Autodesk Fusion 360 part; units mm, degrees
(part 4 of 5)
sketch "Sketch8" plane through (0, 0, 2) normal (0, 0, 1) x (1, 0, 0)
  line L0 (-2.9765, -78.272) -> (-7.3765, -81.7096)
  arc A0 (-9.8, -80.5276) -> (-7.3765, -81.7096) centre (-8.3, -80.5276) ccw
  line L1 (-9.8, -80.5276) -> (-9.8, -73.6105)
  arc A1 (-9.1388, -72.3669) -> (-9.8, -73.6105) centre (-8.3, -73.6105) ccw
  line L2 (-9.1388, -72.3669) -> (-3.9592, -68.8733)
  arc A2 (-2.4, -69.7023) -> (-3.9592, -68.8733) centre (-3.4, -69.7023) ccw
  line L3 (-2.4, -69.7023) -> (-2.4, -77.09)
  arc A3 (-2.9765, -78.272) -> (-2.4, -77.09) centre (-3.9, -77.09) ccw
  line L4 (-2.9765, -60.272) -> (-7.3765, -63.7096)
  arc A4 (-9.8, -62.5276) -> (-7.3765, -63.7096) centre (-8.3, -62.5276) ccw
  line L5 (-9.8, -62.5276) -> (-9.8, -55.6105)
  arc A5 (-9.1388, -54.3669) -> (-9.8, -55.6105) centre (-8.3, -55.6105) ccw
  line L6 (-9.1388, -54.3669) -> (-3.9592, -50.8733)
  arc A6 (-2.4, -51.7023) -> (-3.9592, -50.8733) centre (-3.4, -51.7023) ccw
  line L7 (-2.4, -51.7023) -> (-2.4, -59.09)
  arc A7 (-2.9765, -60.272) -> (-2.4, -59.09) centre (-3.9, -59.09) ccw
  line L8 (7.3765, -81.7096) -> (2.9765, -78.272)
  arc A8 (2.4, -77.09) -> (2.9765, -78.272) centre (3.9, -77.09) ccw
  line L9 (2.4, -77.09) -> (2.4, -69.7023)
  arc A9 (3.9592, -68.8733) -> (2.4, -69.7023) centre (3.4, -69.7023) ccw
  line L10 (3.9592, -68.8733) -> (9.1388, -72.3669)
  arc A10 (9.8, -73.6105) -> (9.1388, -72.3669) centre (8.3, -73.6105) ccw
  line L11 (9.8, -73.6105) -> (9.8, -80.5276)
  arc A11 (7.3765, -81.7096) -> (9.8, -80.5276) centre (8.3, -80.5276) ccw
  line L12 (7.3765, -63.7096) -> (2.9765, -60.272)
  arc A12 (2.4, -59.09) -> (2.9765, -60.272) centre (3.9, -59.09) ccw
  line L13 (2.4, -59.09) -> (2.4, -51.7023)
  arc A13 (3.9592, -50.8733) -> (2.4, -51.7023) centre (3.4, -51.7023) ccw
  line L14 (3.9592, -50.8733) -> (9.1388, -54.3669)
  arc A14 (9.8, -55.6105) -> (9.1388, -54.3669) centre (8.3, -55.6105) ccw
  line L15 (9.8, -55.6105) -> (9.8, -62.5276)
  arc A15 (7.3765, -63.7096) -> (9.8, -62.5276) centre (8.3, -62.5276) ccw
  arc A16 (5.3912, -43.101) -> (4.5193, -42.8216) centre (4.5193, -44.3216) ccw
  line L16 (4.5193, -42.8216) -> (-4.5193, -42.8216)
  arc A17 (-4.5193, -42.8216) -> (-5.3912, -43.101) centre (-4.5193, -44.3216) ccw
  line L17 (-5.3912, -43.101) -> (-6.3588, -43.7922)
  arc A18 (-7.2307, -44.0716) -> (-6.3588, -43.7922) centre (-7.2307, -42.5716) ccw
  line L18 (-7.2307, -44.0716) -> (-7.25, -44.0716)
  arc A19 (-8.75, -42.5716) -> (-7.25, -44.0716) centre (-7.25, -42.5716) ccw
  line L19 (-8.75, -42.5716) -> (-8.75, -35.1771)
  arc A20 (-7.4141, -32.681) -> (-8.75, -35.1771) centre (-5.75, -35.1771) ccw
  line L20 (-7.4141, -32.681) -> (-5.7558, -31.5754)
  arc A21 (-4.0917, -31.0716) -> (-5.7558, -31.5754) centre (-4.0917, -34.0716) ccw
  line L21 (-4.0917, -31.0716) -> (4.0917, -31.0716)
  arc A22 (5.7558, -31.5754) -> (4.0917, -31.0716) centre (4.0917, -34.0716) ccw
  line L22 (5.7558, -31.5754) -> (7.4141, -32.681)
  arc A23 (8.75, -35.1771) -> (7.4141, -32.681) centre (5.75, -35.1771) ccw
  line L23 (8.75, -35.1771) -> (8.75, -42.5716)
  arc A24 (7.25, -44.0716) -> (8.75, -42.5716) centre (7.25, -42.5716) ccw
  line L24 (7.25, -44.0716) -> (7.2307, -44.0716)
  arc A25 (6.3588, -43.7922) -> (7.2307, -44.0716) centre (7.2307, -42.5716) ccw
  line L25 (6.3588, -43.7922) -> (5.3912, -43.101)
  line L26 (-13.75, -77.3) -> (-13.75, -102.3)
  arc A26 (-16.75, -102.3) -> (-13.75, -102.3) centre (-15.25, -102.3) ccw
  line L27 (-16.75, -102.3) -> (-16.75, -77.3)
  arc A27 (-13.75, -77.3) -> (-16.75, -77.3) centre (-15.25, -77.3) ccw
  line L28 (-13.75, -41.5) -> (-13.75, -66.5)
  arc A28 (-16.75, -66.5) -> (-13.75, -66.5) centre (-15.25, -66.5) ccw
  line L29 (-16.75, -66.5) -> (-16.75, -41.5)
  arc A29 (-13.75, -41.5) -> (-16.75, -41.5) centre (-15.25, -41.5) ccw
  line L30 (-13.75, -114.3) -> (-13.75, -139.3)
  arc A30 (-16.75, -139.3) -> (-13.75, -139.3) centre (-15.25, -139.3) ccw
  line L31 (-16.75, -139.3) -> (-16.75, -114.3)
  arc A31 (-13.75, -114.3) -> (-16.75, -114.3) centre (-15.25, -114.3) ccw
  line L32 (16.75, -77.3) -> (16.75, -102.3)
  arc A32 (13.75, -102.3) -> (16.75, -102.3) centre (15.25, -102.3) ccw
  line L33 (13.75, -102.3) -> (13.75, -77.3)
  arc A33 (16.75, -77.3) -> (13.75, -77.3) centre (15.25, -77.3) ccw
  line L34 (13.75, -66.5) -> (13.75, -41.5)
  arc A34 (16.75, -41.5) -> (13.75, -41.5) centre (15.25, -41.5) ccw
  line L35 (16.75, -41.5) -> (16.75, -66.5)
  arc A35 (13.75, -66.5) -> (16.75, -66.5) centre (15.25, -66.5) ccw
  line L36 (13.75, -139.3) -> (13.75, -114.3)
  arc A36 (16.75, -114.3) -> (13.75, -114.3) centre (15.25, -114.3) ccw
  line L37 (16.75, -114.3) -> (16.75, -139.3)
  arc A37 (13.75, -139.3) -> (16.75, -139.3) centre (15.25, -139.3) ccw
  arc A38 (-7.2751, -171.1221) -> (-4.8986, -171.1648) centre (-6.058, -169.5351) ccw
  arc A39 (4.8986, -171.1648) -> (-4.8986, -171.1648) centre (0, -178.05) ccw
  arc A40 (4.8986, -171.1648) -> (7.2751, -171.1221) centre (6.058, -169.5351) ccw
  line L38 (7.2751, -171.1221) -> (15.0344, -165.1715)
  arc A41 (15.0344, -165.1715) -> (16.0278, -163.817) centre (13.2088, -162.7909) ccw
  line L39 (16.0278, -163.817) -> (19.1143, -155.3371)
  arc A42 (19.1143, -155.3371) -> (19.6835, -152.7386) centre (9.7173, -151.9169) ccw
  line L40 (19.6835, -152.7386) -> (20.2399, -145.9914)
  arc A43 (20.2399, -145.9914) -> (20.25, -145.7449) centre (17.25, -145.7449) ccw
  line L41 (20.25, -145.7449) -> (20.25, -35.5)
  arc A44 (20.25, -35.5) -> (19.1875, -32.4184) centre (15.25, -35.5) ccw
  arc A45 (18.55, -30.5695) -> (19.1875, -32.4184) centre (21.55, -30.5695) ccw
  line L42 (18.55, -30.5695) -> (18.55, 0.8857)
  arc A46 (19, 2.4661) -> (18.55, 0.8857) centre (21.55, 0.8857) ccw
  arc A47 (19, 2.4661) -> (9.7944, 5.7648) centre (14.75, 5.1) ccw
  arc A48 (8.9423, 4.0423) -> (9.7944, 5.7648) centre (6.821, 6.1637) ccw
  line L43 (8.9423, 4.0423) -> (1.4142, -3.4858)
  arc A49 (-1.4142, -3.4858) -> (1.4142, -3.4858) centre (0, -2.0716) ccw
  line L44 (-1.4142, -3.4858) -> (-8.9423, 4.0423)
  arc A50 (-9.7944, 5.7648) -> (-8.9423, 4.0423) centre (-6.821, 6.1637) ccw
  arc A51 (-9.7944, 5.7648) -> (-19, 2.4661) centre (-14.75, 5.1) ccw
  arc A52 (-18.55, 0.8857) -> (-19, 2.4661) centre (-21.55, 0.8857) ccw
  line L45 (-18.55, 0.8857) -> (-18.55, -30.5695)
  arc A53 (-19.1875, -32.4184) -> (-18.55, -30.5695) centre (-21.55, -30.5695) ccw
  arc A54 (-19.1875, -32.4184) -> (-20.25, -35.5) centre (-15.25, -35.5) ccw
  line L46 (-20.25, -35.5) -> (-20.25, -145.7449)
  arc A55 (-20.25, -145.7449) -> (-20.2399, -145.9914) centre (-17.25, -145.7449) ccw
  line L47 (-20.2399, -145.9914) -> (-19.6835, -152.7386)
  arc A56 (-19.6835, -152.7386) -> (-19.1143, -155.3371) centre (-9.7173, -151.9169) ccw
  line L48 (-19.1143, -155.3371) -> (-16.0278, -163.817)
  arc A57 (-16.0278, -163.817) -> (-15.0344, -165.1715) centre (-13.2088, -162.7909) ccw
  line L49 (-15.0344, -165.1715) -> (-7.2751, -171.1221)
  arc A58 (4.253, -18.8853) -> (2.35, -19.8578) centre (3.55, -19.8578) ccw
  line L50 (4.253, -18.8853) -> (8.8217, -22.188)
  arc A59 (9.65, -23.8089) -> (8.8217, -22.188) centre (7.65, -23.8089) ccw
  line L51 (9.65, -23.8089) -> (9.65, -25.2396)
  arc A60 (6.43, -26.8244) -> (9.65, -25.2396) centre (7.65, -25.2396) ccw
  line L52 (6.43, -26.8244) -> (2.818, -24.044)
  arc A61 (2.35, -23.0931) -> (2.818, -24.044) centre (3.55, -23.0931) ccw
  line L53 (2.35, -23.0931) -> (2.35, -19.8578)
  circle A62 centre (11.5, -163.1) radius 1.5
  circle A63 centre (-15.25, -108.3) radius 1.5
  arc A64 (-11.75, -14.5) -> (-9.75, -14.5) centre (-10.75, -14.5) ccw
  line L54 (-11.75, -14.5) -> (-11.75, -2.5)
  arc A65 (-9.75, -2.5) -> (-11.75, -2.5) centre (-10.75, -2.5) ccw
  line L55 (-9.75, -2.5) -> (-9.75, -14.5)
  arc A66 (-13.55, -8.5) -> (-15.55, -8.5) centre (-14.55, -8.5) ccw
  line L56 (-13.55, -8.5) -> (-13.55, -20.5)
  arc A67 (-15.55, -20.5) -> (-13.55, -20.5) centre (-14.55, -20.5) ccw
  line L57 (-15.55, -20.5) -> (-15.55, -8.5)
  circle A68 centre (14.75, 5.1) radius 1.5
  circle A69 centre (15.25, -108.3) radius 1.5
  circle A70 centre (-14.75, 5.1) radius 1.5
  arc A71 (15.55, -8.5) -> (13.55, -8.5) centre (14.55, -8.5) ccw
  line L58 (15.55, -8.5) -> (15.55, -20.5)
  arc A72 (13.55, -20.5) -> (15.55, -20.5) centre (14.55, -20.5) ccw
  line L59 (13.55, -20.5) -> (13.55, -8.5)
  arc A73 (-9.65, -25.2396) -> (-6.43, -26.8244) centre (-7.65, -25.2396) ccw
  line L60 (-9.65, -25.2396) -> (-9.65, -23.8089)
  arc A74 (-8.8217, -22.188) -> (-9.65, -23.8089) centre (-7.65, -23.8089) ccw
  line L61 (-8.8217, -22.188) -> (-4.253, -18.8853)
  arc A75 (-2.35, -19.8578) -> (-4.253, -18.8853) centre (-3.55, -19.8578) ccw
  line L62 (-2.35, -19.8578) -> (-2.35, -23.0931)
  arc A76 (-2.818, -24.044) -> (-2.35, -23.0931) centre (-3.55, -23.0931) ccw
  line L63 (-2.818, -24.044) -> (-6.43, -26.8244)
  circle A77 centre (-15.25, -35.5) radius 1.5
  circle A78 centre (15.25, -35.5) radius 1.5
  circle A79 centre (-11.5, -163.1) radius 1.5
  arc A80 (11.75, -2.5) -> (9.75, -2.5) centre (10.75, -2.5) ccw
  line L64 (11.75, -2.5) -> (11.75, -14.5)
  arc A81 (9.75, -14.5) -> (11.75, -14.5) centre (10.75, -14.5) ccw
  line L65 (9.75, -14.5) -> (9.75, -2.5)
  line L66 (-13.75, -85.5776) -> (13.75, -85.5776) construction
  line L67 (8.3, -82.0276) -> (-8.3, -82.0276) construction
  line L68 (8.3, -89.1276) -> (-8.3, -89.1276) construction
  arc A82 (2.4, -101.453) -> (3.9592, -102.282) centre (3.4, -101.453) ccw
  arc A83 (-7.3765, -89.4456) -> (-9.8, -90.6276) centre (-8.3, -90.6276) ccw
  line L69 (-2.4, -101.453) -> (-2.4, -94.0653)
  arc A84 (-9.8, -97.5448) -> (-9.1388, -98.7883) centre (-8.3, -97.5448) ccw
  line L70 (3.9592, -102.282) -> (9.1388, -98.7883)
  arc A85 (2.9765, -92.8833) -> (2.4, -94.0653) centre (3.9, -94.0653) ccw
  arc A86 (9.1388, -98.7883) -> (9.8, -97.5448) centre (8.3, -97.5448) ccw
  line L71 (-2.9765, -92.8833) -> (-7.3765, -89.4456)
  arc A87 (-2.4, -94.0653) -> (-2.9765, -92.8833) centre (-3.9, -94.0653) ccw
  arc A88 (-3.9592, -102.282) -> (-2.4, -101.453) centre (-3.4, -101.453) ccw
  line L72 (7.3765, -89.4456) -> (2.9765, -92.8833)
  arc A89 (9.8, -90.6276) -> (7.3765, -89.4456) centre (8.3, -90.6276) ccw
  line L73 (2.4, -94.0653) -> (2.4, -101.453)
  line L74 (9.8, -97.5448) -> (9.8, -90.6276)
  line L75 (-9.1388, -98.7883) -> (-3.9592, -102.282)
  line L76 (-9.8, -90.6276) -> (-9.8, -97.5448)
  dimension "d75" = 3.55
  constraint coincident L26 L66.start
  constraint coincident L33 L66.end
  constraint perpendicular L33 L66
  constraint coincident A11 L67.start
  constraint coincident A0 L67.end
  constraint tangent A0 L67
  constraint tangent A11 L67
  constraint symmetric L0.start L66 L71.start
  constraint symmetric L0.end L66 A83.start
  constraint symmetric A0.start L66 A83.end
  constraint symmetric A0 L66 A83
  constraint symmetric L1.end L66 A84.start
  constraint symmetric A1.start L66 A84.end
  constraint symmetric A1 L66 A84
  constraint symmetric L2.end L66 A88.start
  constraint symmetric A2.start L66 L69.start
  constraint symmetric A2 L66 A88
  constraint symmetric L3.end L66 L69.end
  constraint symmetric A3 L66 A87
  constraint symmetric L8.start L66 L72.start
  constraint symmetric L8.end L66 A85.start
  constraint symmetric A8.start L66 A85.end
  constraint symmetric A8 L66 A85
  constraint symmetric L9.end L66 A82.start
  constraint symmetric A9.start L66 A82.end
  constraint symmetric A9 L66 A82
  constraint symmetric L10.end L66 L70.end
  constraint symmetric A10.start L66 A86.end
  constraint symmetric A10 L66 A86
  constraint symmetric L11.end L66 A89.start
  constraint symmetric A11 L66 A89
  constraint symmetric L66 L67.start L68.start
  constraint symmetric L66 L67.end L68.end
  measures "d75" distance of L66 L67
extrude "Extrude5" cut sketch "Sketch8" against normal blind 2 contours A82 L70 A85 A86 L72 A89 L73 L74 | A83 L69 A84 L71 A87 A88 L75 L76
pattern_linear "R-Pattern2" count 4 spacing 18 along (0, -1, 0) of "Extrude5"
equation "d35 = ( 17.5 / 2 ) * 1 mm"
equation "d54 = ( 4.8 / 2 ) * 1 mm"
equation "d75 = ( 7.1 / 2 ) * 1 mm"

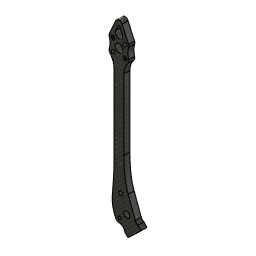
design "arm_rear_6mm"
Autodesk Fusion 360 part; units mm, degrees
sketch "Sketch1" plane through (0, 0, 0) normal (0, 0, 1) x (1, 0, 0)
  circle A0 centre (0, 0) radius 3.95
  line L0 (0, 0) -> (0, -178.3291)
  line L1 (-5, 0) -> (-5, -178.3291)
  line L2 (5, 0) -> (5, -178.3291)
  dimension "d1" = 7.9
  dimension "d2" = 5
  dimension "d3" = -5
  constraint coincident A0.centre L0.start
  constraint vertical L0
  measures "d1" diameter of A0
sketch "Sketch2" plane through (0, 0, 0) normal (0, 0, 1) x (1, 0, 0)
  circle A0 centre (0, 0) radius 3.95
  line L0 (0, 0) -> (-9, 0) construction
  line L1 (7.566, -7.566) -> (4.5962, -4.5962) construction
  line L2 (6.7175, 4.5962) -> (7.566, 5.4447)
  line L3 (4.5962, -6.7175) -> (5.4447, -7.566)
  line L4 (0.9091, 19.0167) -> (3.409, 13.5625)
  circle A1 centre (6.5054, -6.5054) radius 3.5
  line L5 (-4.5962, 6.7175) -> (-5.4447, 7.566)
  arc A2 (4.5962, 6.7175) -> (6.7175, 4.5962) centre (5.6569, 5.6569) ccw
  arc A3 (-7.566, -5.4447) -> (-5.4447, -7.566) centre (-6.5054, -6.5054) ccw
  arc A4 (9.1588, -8.7878) -> (5, -20) centre (22.1936, -20) ccw
  line L6 (7.566, -5.4447) -> (6.7175, -4.5962)
  arc A5 (9.8421, 5.4488) -> (9.8421, -5.4488) centre (27.0494, 0) ccw
  arc A6 (-4.5962, -6.7175) -> (-6.7175, -4.5962) centre (-5.6569, -5.6569) ccw
  circle A7 centre (0, 21) radius 3.5
  circle A8 centre (0, 12) radius 3.75
  line L7 (-5, -20) -> (5, -20) construction
  line L8 (-0.9091, 19.0167) -> (-3.409, 13.5625)
  arc A9 (5.4447, -7.566) -> (7.566, -5.4447) centre (6.5054, -6.5054) ccw
  line L9 (-6.7175, -4.5962) -> (-7.566, -5.4447)
  arc A10 (-5, -20) -> (-9.1588, -8.7878) centre (-22.1936, -20) ccw
  line L10 (5.4447, 7.566) -> (4.5962, 6.7175)
  line L11 (0, 0) -> (18.7579, 0) construction
  circle A11 centre (-6.5054, -6.5054) radius 3.5
  line L12 (-9.6985, 7.9385) -> (-3.1931, 22.4331)
  arc A12 (6.7175, -4.5962) -> (4.5962, -6.7175) centre (5.6569, -5.6569) ccw
  arc A13 (7.566, 5.4447) -> (5.4447, 7.566) centre (6.5054, 6.5054) ccw
  circle A14 centre (-6.5054, 6.5054) radius 3.5
  line L13 (0, 0) -> (13.2638, -13.2638) construction
  line L14 (0, 24.5) -> (0, 0) construction
  line L15 (9.6985, 7.9385) -> (3.1931, 22.4331)
  arc A15 (-6.7175, 4.5962) -> (-4.5962, 6.7175) centre (-5.6569, 5.6569) ccw
  line L16 (-5.4447, -7.566) -> (-4.5962, -6.7175)
  line L17 (-7.566, 5.4447) -> (-6.7175, 4.5962)
  arc A16 (-5.4447, 7.566) -> (-7.566, 5.4447) centre (-6.5054, 6.5054) ccw
  arc A17 (-9.8421, -5.4488) -> (-9.8421, 5.4488) centre (-27.0494, 0) ccw
  circle A18 centre (6.5054, 6.5054) radius 3.5
  arc A19 (0.9091, 19.0167) -> (-0.9091, 19.0167) centre (0, 18.6) ccw
  arc A20 (16.4975, -142.4127) -> (19.1132, -145.1691) centre (20.2426, -141.4781) ccw
  circle A21 centre (28.5466, -163.0999) radius 2.95 construction
  line L18 (36.8072, -178.2122) -> (44.0178, -178.0032) construction
  line L19 (-6.1772, -125.1087) -> (-6.7634, -132.2985)
  line L20 (0.7848, -157.6755) -> (0.9047, -157.0861) construction
  arc A22 (12.4548, -169.2574) -> (12.1429, -164.1911) centre (12.0783, -166.7378) ccw construction
  circle A23 centre (0.6152, -147.9032) radius 1.5
  line L21 (5.9477, -157.6628) -> (12.1429, -164.1911)
  arc A24 (5.9477, -157.6628) -> (0.9047, -157.0861) centre (3.4011, -157.594) ccw
  arc A25 (-7.3343, -135.681) -> (-6.7634, -132.2985) centre (-26.6972, -130.6734) ccw construction
  arc A26 (10.3319, -168.8201) -> (11.86, -169.3463) centre (11.6013, -167.6155) ccw construction
  arc A27 (44.0178, -178.0032) -> (46.9539, -162.6605) centre (43.7859, -170.0066) ccw construction
  arc A28 (36.8072, -178.2122) -> (33.3994, -178.6053) centre (37.3868, -198.2038) ccw construction
  arc A29 (9.2981, -122.9795) -> (-6.1772, -125.1087) centre (1.7963, -125.7587) ccw construction
  line L22 (-7.3343, -135.681) -> (-10.3423, -147.312) construction
  circle A30 centre (21.61, -170.0271) radius 1.5 construction
  line L23 (21.627, -181.0005) -> (33.3994, -178.6053) construction
  arc A31 (0.7848, -157.6755) -> (1.2303, -159.229) centre (2.4997, -158.0244) ccw construction
  line L24 (46.9539, -162.6605) -> (27.9242, -154.4539) construction
  circle A32 centre (1.7963, -125.7587) radius 2
  line L25 (10.3319, -168.8201) -> (1.2303, -159.229) construction
  line L26 (12.4548, -169.2574) -> (11.86, -169.3463) construction
  circle A33 centre (43.7859, -170.0066) radius 2 construction
  line L27 (25.3084, -151.6975) -> (19.1132, -145.1691)
  line L28 (16.4975, -142.4127) -> (9.2981, -122.9795)
  arc A34 (25.3084, -151.6975) -> (27.9242, -154.4539) centre (29.0536, -150.7628) ccw construction
  circle A35 centre (7.8959, -141.3387) radius 2.95
  circle A36 centre (0.6152, -147.9032) radius 4.5
  spline S0 degree 5 poles (0.6152, -152.4032) (0.9218, -152.4032) (1.5117, -152.4518) (2.3269, -152.6706) (3.2887, -153.2145) (4.3168, -154.1801) (5.002, -155.1015) (5.4252, -155.8554) (5.6626, -156.3853) (5.77, -156.657) knots 0 0 0 0 0 0 0.2 0.4 0.6 0.8 1 1 1 1 1 1
  line L29 (22.2108, -148.4333) -> (9.0453, -160.927)
  spline S1 degree 5 poles (-6.7634, -132.2985) (-6.8228, -133.0274) (-6.8958, -134.4803) (-6.8677, -136.6451) (-6.5849, -139.5032) (-5.9007, -143.0251) (-5.105, -145.7887) (-4.35, -147.8195) (-3.7693, -149.1519) (-3.4595, -149.8128) knots 0 0 0 0 0 0 0.2 0.4 0.6 0.8 1 1 1 1 1 1
  line L30 (0, 0) -> (0, -133.0837) construction
  line L31 (-5, 0) -> (-5, -133.0837)
  line L32 (5, 0) -> (5, -133.0837)
  spline S2 degree 5 poles (-6.1772, -125.1087) (-6.1092, -124.2742) (-5.9743, -122.6052) (-5.7752, -120.101) (-5.5198, -116.7611) (-5.2405, -112.5839) (-5.0796, -109.2394) (-5.0145, -106.7287) (-5, -105.0538) (-5, -104.2161) knots 0 0 0 0 0 0 0.2 0.4 0.6 0.8 1 1 1 1 1 1
  spline S3 degree 5 poles (9.2981, -122.9795) (8.8487, -121.7665) (8.0283, -119.3245) (7.033, -115.6132) (6.1133, -110.5828) (5.4305, -104.2105) (5.1351, -99.0813) (5.0246, -95.2302) (5, -92.6623) (5, -91.3783) knots 0 0 0 0 0 0 0.2 0.4 0.6 0.8 1 1 1 1 1 1
  point P0 (0, 24.5)
  dimension "d5" = 360
  dimension "d6" = 45
  dimension "d7" = 3
  dimension "d8" = 6.5
  dimension "d9" = 4.2
  dimension "d10" = 7
  dimension "d11" = 24.5
  dimension "d12" = 7
  dimension "d13" = 7
  dimension "d14" = 9
  dimension "d15" = 20
  dimension "d16" = 7.5
  dimension "d17" = 12
  dimension "d18" = 1
  dimension "d19" = 9
  dimension "d20" = 5
  dimension "d21" = -5
  constraint horizontal L11
  constraint coincident A0.centre L0.start
  constraint tangent L6 A12
  constraint tangent L3 A12
  constraint parallel L3 L6
  constraint tangent L3 A9
  constraint tangent L6 A9
  constraint midpoint L1.start A9
  constraint midpoint L1.end A12
  constraint coincident L1.end L13
  constraint parallel L1 L13
  constraint coincident P0 L14.start
  constraint perpendicular L11 L14
  constraint coincident P0 A7
  constraint concentric A14 A16
  constraint concentric A3 A11
  constraint perpendicular L0 L14
  constraint coincident L0.end A17
  constraint coincident A17.end A14
  constraint coincident A17.start A11
  constraint tangent A14 A17
  constraint tangent A11 A17
  constraint horizontal L7
  constraint tangent A10 A11
  constraint coincident A10.end A11
  constraint coincident A7.centre L14
  constraint coincident L12.start A14
  constraint coincident L12.end A7
  constraint tangent A7 L12
  constraint tangent L12 A14
  constraint symmetric L7.start A4.end L14
  constraint symmetric A14 L14 A18
  constraint symmetric A17.start A5.end L14
  constraint symmetric A17.end A5.start L14
  constraint symmetric A5 L14 A17
  constraint symmetric A10.end A4.start L14
  constraint symmetric A4 A10 L14
  constraint symmetric L12.start L15.start L14
  constraint symmetric L12.end L15.end L14
  constraint symmetric A1 A11 L14
  constraint coincident A8.centre L14
  constraint coincident L4.end A8
  constraint tangent L4 A8
  constraint coincident L8.end A8
  constraint tangent A8 L8
  constraint tangent L4 A19
  constraint tangent L8 A19
  constraint concentric A23 A36
  constraint coincident A36 S0.start
  constraint coincident A24 S0.end
  constraint tangent A24 S0
  constraint tangent A36 S0
  constraint midpoint L27 L29.start
  constraint midpoint L21 L29.end
  constraint coincident A36 S1.end
  constraint tangent A36 S1
  constraint perpendicular L7 L30
  constraint coincident L31 S2.end
  constraint coincident L32 S3.end
  measures "d6" angle of L11 L13
  measures "d7" diameter of A12
  measures "d8" distance of A0.centre L1.end
  measures "d9" distance of L1.start L1.end
  measures "d10" diameter of A7
  measures "d11" distance of P0 A0.centre
  measures "d12" diameter of A14
  measures "d13" diameter of A11
  measures "d14" distance of L0.end A0.centre
  measures "d15" distance of A0.centre L7
  measures "d16" diameter of A8
  measures "d17" distance of A8.centre A0.centre
  measures "d18" radius of A19
  measures "d19" diameter of A36
extrude "Extrude1" add sketch "Sketch2" along normal blind 6 contours L3 A1 A12 L32 | L3 A1 L6 A9 A12 L32 | L4 A1 A5 A7 A8 L8 A11 L12 A14 L15 A17 A18 A20 L19 L21 A24 L27 L28 A36 S0 L29 S1 L31 L32 S2 S3 | A1 A4 L32 | A18 | L4 A7 L8 A19 | A14 | A3 A6 L9 A11 L16 L31 | A10 A11 L31 | A6 A11 L16 L31 | A36 picked at (0.167, 22.8547)

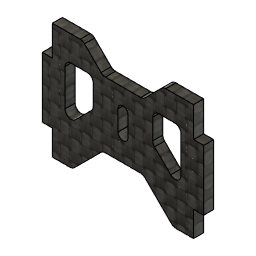
design "cam_mount_2mm"
Autodesk Fusion 360 part; units mm, degrees
sketch "Sketch1" plane through (0, 0, 0) normal (0, 0, 1) x (1, 0, 0)
  line L0 (-16, 11.5) -> (16, 11.5)
  line L1 (16, 11.5) -> (16, -11.5)
  line L2 (16, -11.5) -> (-16, -11.5)
  line L3 (-16, -11.5) -> (-16, 11.5)
  line L4 (-16, 11.5) -> (16, -11.5) construction
  line L5 (16, 11.5) -> (-16, -11.5) construction
  dimension "d1" = 32
  dimension "d2" = 23
  constraint horizontal L0
  constraint perpendicular L0 L1
  constraint parallel L0 L2
  constraint parallel L1 L3
  constraint coincident L4 origin
  constraint coincident L5 origin
  measures "d1" distance of L1.end L2.end
  measures "d2" distance of L0.end L1.end
sketch "Sketch2" plane through (0, 0, 0) normal (0, 0, 1) x (1, 0, 0)
  line L0 (-14, 11.5) -> (14, 11.5)
  line L1 (14, 11.5) -> (14, -11.5)
  line L2 (14, -11.5) -> (-14, -11.5)
  line L3 (-14, -11.5) -> (-14, 11.5)
  line L4 (-14, 11.5) -> (14, -11.5) construction
  line L5 (14, 11.5) -> (-14, -11.5) construction
  line L6 (-16, 5.5) -> (-14, 5.5)
  line L7 (-14, 5.5) -> (-14, -6.5)
  line L8 (-14, -6.5) -> (-16, -6.5)
  line L9 (-16, -6.5) -> (-16, 5.5)
  line L10 (-16, -11.5) -> (-16, 11.5)
  line L11 (-4, 7.5) -> (4, 7.5)
  line L12 (-16, 11.5) -> (16, 11.5)
  line L13 (-4, 7.5) -> (-8, 11.5)
  line L14 (-4, 7.5) -> (0.1526, 7.5) construction
  line L15 (4, 7.5) -> (8, 11.5)
  line L16 (4, 7.5) -> (8.8443, 7.5) construction
  line L17 (0, 0) -> (0, 17.5574) construction
  line L18 (-4, -5.5) -> (4, -5.5)
  line L19 (-4, -5.5) -> (-10, -11.5)
  line L20 (-4, -5.5) -> (4.4853, -5.5) construction
  line L21 (4, -5.5) -> (10, -11.5)
  line L22 (14, 5.5) -> (16, 5.5)
  line L23 (16, 5.5) -> (16, -6.5)
  line L24 (16, -6.5) -> (14, -6.5)
  line L25 (14, -6.5) -> (14, 5.5)
  line L26 (16, 11.5) -> (16, -11.5)
  line L27 (-1, 3.3) -> (-1, -0.7)
  arc A0 (-1, -0.7) -> (1, -0.7) centre (0, -0.7) ccw
  line L28 (1, -0.7) -> (1, 3.3)
  arc A1 (1, 3.3) -> (-1, 3.3) centre (0, 3.3) ccw
  line L29 (0, 4.3) -> (0, -1.7) construction
  line L30 (11.5, 6.5) -> (5.9, 6.5)
  line L31 (5.9, 6.5) -> (5.9, -2.8)
  line L32 (5.9, -2.8) -> (11.5, -2.8)
  line L33 (11.5, -2.8) -> (11.5, 6.5)
  line L34 (5.9, 0.7355) -> (9.4355, -2.8)
  line L35 (5.9, 0.7355) -> (4.4836, 0.7355) construction
  line L36 (11.5, -2.8) -> (11.5, -4.8645)
  line L37 (11.5, -4.8645) -> (9.4355, -2.8)
  point P0 (0, 7.5)
  dimension "d3" = 28
  dimension "d4" = 23
  dimension "d5" = 12
  dimension "d6" = 4
  dimension "d7" = 135
  dimension "d8" = 45
  dimension "d9" = 8
  dimension "d10" = 13
  dimension "d11" = 135
  dimension "d12" = 90
  dimension "d13" = 6
  dimension "d14" = 12
  dimension "d15" = 6
  dimension "d16" = 2
  dimension "d17" = 6
  dimension "d18" = 3.8
  dimension "d19" = 5.6
  dimension "d20" = 9.3
  dimension "d21" = 2.5
  dimension "d22" = 1
  dimension "d23" = 45
  dimension "d24" = 5
  constraint horizontal L0
  constraint perpendicular L0 L1
  constraint parallel L0 L2
  constraint parallel L1 L3
  constraint coincident L4 L17.start
  constraint coincident L5 L17.start
  constraint coincident L17.start origin
  constraint horizontal L6
  constraint vertical L7
  constraint horizontal L8
  constraint vertical L9
  constraint coincident L3 L7.end
  constraint coincident L6.start L10
  constraint horizontal L11
  constraint horizontal L14
  constraint coincident L0 L13.end
  constraint horizontal L16
  constraint coincident L0 L15.end
  constraint vertical L17
  constraint midpoint L11 P0
  constraint coincident L17 P0
  constraint horizontal L20
  constraint coincident L2 L19.end
  constraint coincident L2 L21.end
  constraint horizontal L22
  constraint vertical L23
  constraint horizontal L24
  constraint vertical L25
  constraint coincident L1 L22.start
  constraint coincident L22.end L26
  constraint tangent L27 A0
  constraint tangent A0 L28
  constraint parallel L27 L28
  constraint tangent L28 A1
  constraint tangent L27 A1
  constraint midpoint A1 L29.start
  constraint midpoint A0 L29.end
  constraint parallel L17 L29
  constraint coincident L17 L29.start
  constraint horizontal L30
  constraint vertical L31
  constraint horizontal L32
  constraint vertical L33
  constraint horizontal L35
  constraint coincident L31 L34.start
  constraint coincident L32 L34.end
  constraint perpendicular L32 L36
  constraint parallel L34 L37
  measures "d3" distance of L1.end L2.end
  measures "d4" distance of L0.end L1.end
  measures "d5" distance of L6 L8
  measures "d6" distance of L11 L12
  measures "d7" angle of L13 L14
  measures "d8" angle of L15 L16
  measures "d9" distance of L11.start L11.end
  measures "d11" angle of L19 L20
  measures "d12" angle of L19 L21
  measures "d13" distance of L6 L12
  measures "d14" distance of L22.start L24.end
  measures "d15" distance of L12 L22
  measures "d16" diameter of A0
  measures "d17" distance of L29.start L29.end
  measures "d18" distance of L20 L29.end
  measures "d19" distance of L30.start L30.end
  measures "d20" distance of L30.start L32.end
  measures "d21" distance of L25 L33
  measures "d22" distance of L11 L30
  measures "d23" angle of L34 L35
  measures "d24" distance of L34.start L34.end
extrude "Extrude1" add sketch "Sketch2" along normal blind 2 contours L0 L1 L2 L3 L7 L11 L12 L13 L15 L18 L19 L21 L25 | L3 L6 L7 L8 L9 L10 | L1 L22 L23 L24 L25 L26 | L30 L31 L32 L33 L34 | L32 L36 L37 | L31 L32 L34
extrude "Extrude2" cut sketch "Sketch2" along normal blind 5 contours L30 L31 L32 L33 L34 | L32 L36 L37
fillet "Fillet1" radius 1.2 4 edges at (11.5, -4.8645, 1) (5.9, 0.7355, 1) (5.9, 6.5, 1) (11.5, 6.5, 1)
mirror "Mirror1" about plane through (0, 0, 0) normal (1, 0, 0) of "Extrude2", "Fillet1"
fillet "Fillet2" radius 1.2 8 edges at (-4, -5.5, 1) (-10, -11.5, 1) (4, -5.5, 1) (10, -11.5, 1) (-8, 11.5, 1) (-4, 7.5, 1) (4, 7.5, 1) (8, 11.5, 1)

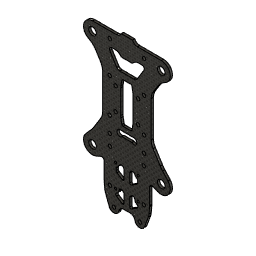
design "mid_plate_2mm"
Autodesk Fusion 360 part; units mm, degrees
sketch "Sketch1" plane through (0, 0, 0) normal (0, 0, 1) x (1, 0, 0)
  line L0 (21.55, -50.4796) -> (21.55, -18.7607)
  line L1 (-21.55, -18.7607) -> (-21.55, -50.4796)
  circle A0 centre (15.25, -19.35) radius 2.95 construction
  circle A1 centre (-15.25, -19.35) radius 2.95 construction
  arc A2 (10.3384, 3) -> (6.0958, 1.2426) centre (10.3384, -3) ccw
  line L2 (-27.7114, -5.7461) -> (-23.2215, -12.9316)
  line L3 (29.5877, -66.4969) -> (23.2215, -56.3087)
  arc A3 (21.55, -50.4796) -> (23.2215, -56.3087) centre (32.55, -50.4796) ccw
  line L4 (4.8532, 0) -> (6.0958, 1.2426)
  circle A4 centre (15, -73.65) radius 2.95 construction
  arc A5 (4.5, -61) -> (8.3897, -57.7389) centre (6.3028, -59.2001) ccw
  line L5 (30.5, 15.05) -> (21.55, 15.05)
  arc A6 (8.0447, -57.2462) -> (6.6112, -56.5) centre (6.6112, -58.25) ccw
  line L6 (-4.5, -79.15) -> (4.5, -79.15) construction
  circle A7 centre (30.5, -79.95) radius 2 construction
  circle A8 centre (15.25, -49.85) radius 2.95 construction
  arc A9 (27.3521, -87.3046) -> (36.4601, -74.6136) centre (30.5, -79.95) ccw
  arc A10 (-8.3897, -57.7389) -> (-4.5, -61) centre (-6.3028, -59.2001) ccw
  arc A11 (-30.5, 15.05) -> (-33.9547, -0.1656) centre (-30.5, 7.05) ccw
  arc A12 (-6.0958, 1.2426) -> (-10.3384, 3) centre (-10.3384, -3) ccw
  line L7 (-27.3521, -87.3046) -> (-20.2, -84.2434)
  arc A13 (-31.6483, -69.2394) -> (-29.5877, -66.4969) centre (-46.5487, -55.8985) ccw
  line L8 (-13.5, 3) -> (-10.3384, 3)
  line L9 (-6.0958, 1.2426) -> (-4.8532, 0)
  line L10 (-31.6483, -69.2394) -> (-36.4601, -74.6136)
  arc A14 (15.1961, -0.0598) -> (13.5, 3) centre (13.5, 1) ccw
  arc A15 (19, 46.9161) -> (14.75, 54.55) centre (14.75, 49.55) ccw construction
  arc A16 (-36.4601, -74.6136) -> (-27.3521, -87.3046) centre (-30.5, -79.95) ccw
  circle A17 centre (-15.25, -49.85) radius 2.95 construction
  arc A18 (-6.6112, -56.5) -> (-8.0447, -57.2462) centre (-6.6112, -58.25) ccw
  line L11 (0.3197, 52.9873) -> (5.4482, 50.7517) construction
  arc A19 (2.7973, 58.6708) -> (-2.7973, 58.6708) centre (0, 52.254) ccw construction
  circle A20 centre (-15, -73.65) radius 2.95 construction
  line L12 (-23.2215, -56.3087) -> (-29.5877, -66.4969)
  arc A21 (18.55, 18.05) -> (21.55, 15.05) centre (21.55, 18.05) ccw construction
  arc A22 (-1.3481, 45.8161) -> (1.3481, 45.8161) centre (0, 47.9215) ccw construction
  arc A23 (33.9547, -0.1656) -> (30.5, 15.05) centre (30.5, 7.05) ccw
  line L13 (6.189, -12.7) -> (-6.189, -12.7) construction
  arc A24 (-13.5, 3) -> (-15.1961, -0.0598) centre (-13.5, 1) ccw
  circle A25 centre (15.25, -63.85) radius 1.5
  arc A26 (8.3, -79.15) -> (4.5, -79.15) centre (6.4, -82.51) ccw construction
  circle A27 centre (15.25, 8.95) radius 1.5
  circle A28 centre (-30.5, 7.05) radius 2 construction
  arc A29 (7.55, 40.0871) -> (5.7029, 41.0977) centre (6.35, 40.0871) ccw construction
  arc A30 (9.75, 29.95) -> (11.75, 29.95) centre (10.75, 29.95) ccw construction
  arc A31 (2.35, 33.9294) -> (3.3622, 32.0776) centre (4.55, 33.9294) ccw construction
  line L14 (10.9121, 55.1332) -> (2.7973, 58.6708) construction
  line L15 (-5.4482, 50.7517) -> (-0.3197, 52.9873) construction
  line L16 (9.75, 29.95) -> (9.75, 41.95) construction
  arc A32 (-13.7095, 54.55) -> (-10.9121, 55.1332) centre (-13.7095, 61.55) ccw construction
  line L17 (4.253, 25.5647) -> (8.8217, 22.262) construction
  line L18 (14.75, 54.55) -> (13.7095, 54.55) construction
  line L19 (6.43, 17.6256) -> (2.818, 20.406) construction
  line L20 (-2.7973, 58.6708) -> (-10.9121, 55.1332) construction
  circle A33 centre (-14.75, 49.55) radius 1.5 construction
  line L21 (9.65, 20.6411) -> (9.65, 19.2104) construction
  line L22 (2.35, 33.9294) -> (2.35, 37.7471) construction
  arc A34 (3.3637, 39.5999) -> (2.35, 37.7471) centre (4.55, 37.7471) ccw construction
  line L23 (-8.8217, 22.262) -> (-4.253, 25.5647) construction
  arc A35 (11.75, 41.95) -> (9.75, 41.95) centre (10.75, 41.95) ccw construction
  arc A36 (-13.55, 35.95) -> (-15.55, 35.95) centre (-14.55, 35.95) ccw construction
  line L24 (18.55, 18.05) -> (18.55, 45.3357) construction
  line L25 (-2.35, 24.5922) -> (-2.35, 21.3569) construction
  line L26 (13.55, 23.95) -> (13.55, 35.95) construction
  arc A37 (15.55, 35.95) -> (13.55, 35.95) centre (14.55, 35.95) ccw construction
  circle A38 centre (14.75, 49.55) radius 1.5 construction
  arc A39 (-2.818, 20.406) -> (-2.35, 21.3569) centre (-3.55, 21.3569) ccw construction
  line L27 (7.55, 40.0871) -> (7.55, 33.4162) construction
  arc A40 (5.6227, 48.5531) -> (5.4482, 50.7517) centre (4.9486, 49.6058) ccw construction
  arc A41 (-2.35, 37.7471) -> (-3.3637, 39.5999) centre (-4.55, 37.7471) ccw construction
  arc A42 (-3.3622, 32.0776) -> (-2.35, 33.9294) centre (-4.55, 33.9294) ccw construction
  arc A43 (4.1622, 31.5645) -> (7.55, 33.4162) centre (5.35, 33.4162) ccw construction
  line L28 (-11.75, 29.95) -> (-11.75, 41.95) construction
  line L29 (-2.818, 20.406) -> (-6.43, 17.6256) construction
  line L30 (-9.75, 41.95) -> (-9.75, 29.95) construction
  line L31 (4.1622, 31.5645) -> (3.3622, 32.0776) construction
  arc A44 (-14.75, 54.55) -> (-19, 46.9161) centre (-14.75, 49.55) ccw construction
  line L32 (11.75, 41.95) -> (11.75, 29.95) construction
  line L33 (-13.7095, 54.55) -> (-14.75, 54.55) construction
  line L34 (-15.55, 23.95) -> (-15.55, 35.95) construction
  arc A45 (-15.55, 23.95) -> (-13.55, 23.95) centre (-14.55, 23.95) ccw construction
  line L35 (5.6227, 48.5531) -> (1.3481, 45.8161) construction
  arc A46 (-7.55, 33.4162) -> (-4.1622, 31.5645) centre (-5.35, 33.4162) ccw construction
  line L36 (-9.65, 19.2104) -> (-9.65, 20.6411) construction
  arc A47 (-2.35, 24.5922) -> (-4.253, 25.5647) centre (-3.55, 24.5922) ccw construction
  line L37 (-1.3481, 45.8161) -> (-5.6227, 48.5531) construction
  arc A48 (-5.7029, 41.0977) -> (-7.55, 40.0871) centre (-6.35, 40.0871) ccw construction
  arc A49 (-18.55, 45.3357) -> (-19, 46.9161) centre (-21.55, 45.3357) ccw construction
  line L38 (-3.3622, 32.0776) -> (-4.1622, 31.5645) construction
  arc A50 (4.253, 25.5647) -> (2.35, 24.5922) centre (3.55, 24.5922) ccw construction
  arc A51 (0.3197, 52.9873) -> (-0.3197, 52.9873) centre (0, 52.254) ccw construction
  arc A52 (19, 46.9161) -> (18.55, 45.3357) centre (21.55, 45.3357) ccw construction
  line L39 (2.35, 21.3569) -> (2.35, 24.5922) construction
  arc A53 (10.9121, 55.1332) -> (13.7095, 54.55) centre (13.7095, 61.55) ccw construction
  line L40 (-13.55, 35.95) -> (-13.55, 23.95) construction
  arc A54 (13.55, 23.95) -> (15.55, 23.95) centre (14.55, 23.95) ccw construction
  line L41 (-2.35, 37.7471) -> (-2.35, 33.9294) construction
  line L42 (-7.55, 33.4162) -> (-7.55, 40.0871) construction
  arc A55 (9.65, 20.6411) -> (8.8217, 22.262) centre (7.65, 20.6411) ccw construction
  arc A56 (-5.4482, 50.7517) -> (-5.6227, 48.5531) centre (-4.9486, 49.6058) ccw construction
  arc A57 (2.35, 21.3569) -> (2.818, 20.406) centre (3.55, 21.3569) ccw construction
  arc A58 (-8.8217, 22.262) -> (-9.65, 20.6411) centre (-7.65, 20.6411) ccw construction
  line L43 (-5.7029, 41.0977) -> (-3.3637, 39.5999) construction
  line L44 (3.3637, 39.5999) -> (5.7029, 41.0977) construction
  line L45 (-18.55, 45.3357) -> (-18.55, 18.05) construction
  line L46 (15.55, 35.95) -> (15.55, 23.95) construction
  arc A59 (-9.75, 41.95) -> (-11.75, 41.95) centre (-10.75, 41.95) ccw construction
  arc A60 (-11.75, 29.95) -> (-9.75, 29.95) centre (-10.75, 29.95) ccw construction
  line L47 (4.5, -61) -> (-4.5, -61)
  arc A61 (6.43, 17.6256) -> (9.65, 19.2104) centre (7.65, 19.2104) ccw construction
  arc A62 (-9.65, 19.2104) -> (-6.43, 17.6256) centre (-7.65, 19.2104) ccw construction
  line L48 (36.4601, -74.6136) -> (31.6483, -69.2394)
  arc A63 (-21.55, 15.05) -> (-18.55, 18.05) centre (-21.55, 18.05) ccw construction
  line L49 (-6.6112, -56.5) -> (6.6112, -56.5)
  line L50 (-21.55, 15.05) -> (-30.5, 15.05)
  line L51 (8.0447, -57.2462) -> (8.3897, -57.7389)
  circle A64 centre (-15.25, 8.95) radius 1.5
  line L52 (8.3, -79.15) -> (27.3521, -87.3046) construction
  arc A65 (29.5877, -66.4969) -> (31.6483, -69.2394) centre (46.5487, -55.8985) ccw
  circle A66 centre (-30.5, -79.95) radius 2 construction
  line L53 (-8.3897, -57.7389) -> (-8.0447, -57.2462)
  arc A67 (-27.7114, -5.7461) -> (-33.9547, -0.1656) centre (-40.4322, -13.6949) ccw
  line L54 (10.3384, 3) -> (13.5, 3)
  arc A68 (23.2215, -12.9316) -> (21.55, -18.7607) centre (32.55, -18.7607) ccw
  arc A69 (-23.2215, -56.3087) -> (-21.55, -50.4796) centre (-32.55, -50.4796) ccw
  arc A70 (-4.5, -79.15) -> (-8.3, -79.15) centre (-6.4, -82.51) ccw construction
  arc A71 (33.9547, -0.1656) -> (27.7114, -5.7461) centre (40.4322, -13.6949) ccw
  arc A72 (-21.55, -18.7607) -> (-23.2215, -12.9316) centre (-32.55, -18.7607) ccw
  circle A73 centre (30.5, 7.05) radius 2 construction
  circle A74 centre (-15.25, -63.85) radius 1.5
  line L55 (-4.8532, 0) -> (4.8532, 0)
  line L56 (23.2215, -12.9316) -> (27.7114, -5.7461)
  line L57 (15.1961, -0.0598) -> (9.0119, -10.0491)
  circle A75 centre (-30.5, 7.05) radius 3.375
  circle A76 centre (30.5, 7.05) radius 3.375
  circle A77 centre (-30.5, -79.95) radius 3.375
  circle A78 centre (30.5, -79.95) radius 3.375
  circle A79 centre (-15.25, -19.35) radius 1.5
  circle A80 centre (15.25, -19.35) radius 1.5
  circle A81 centre (15.25, -49.85) radius 1.5
  circle A82 centre (-15.25, -49.85) radius 1.5
  line L58 (-15.25, -19.35) -> (15.25, -49.85) construction
  line L59 (-10, -24.6) -> (10, -24.6) construction
  line L60 (10, -24.6) -> (10, -44.6) construction
  line L61 (10, -44.6) -> (-10, -44.6) construction
  line L62 (-10, -44.6) -> (-10, -24.6) construction
  line L63 (-10, -24.6) -> (10, -44.6) construction
  line L64 (10, -24.6) -> (-10, -44.6) construction
  circle A83 centre (-10, -24.6) radius 1.5
  circle A84 centre (10, -24.6) radius 1.5
  circle A85 centre (10, -44.6) radius 1.5
  circle A86 centre (-10, -44.6) radius 1.5
  circle A87 centre (-15, -73.65) radius 1.5
  circle A88 centre (15, -73.65) radius 1.5
  line L65 (6.189, -11.4) -> (-6.189, -11.4)
  line L66 (0, 44.45) -> (0, -156.9165) construction
  spline S0 degree 5 poles (9.0119, -10.0491) (8.9382, -10.1683) (8.7794, -10.3902) (8.5077, -10.6735) (8.0875, -10.964) (7.4965, -11.2156) (6.9894, -11.3405) (6.5947, -11.3892) (6.3253, -11.4) (6.189, -11.4) knots 0 0 0 0 0 0 0.2 0.4 0.6 0.8 1 1 1 1 1 1
  line L67 (-15.1961, -0.0598) -> (-9.0119, -10.0491)
  spline S1 degree 5 poles (-9.0119, -10.0491) (-8.9382, -10.1683) (-8.7794, -10.3902) (-8.5077, -10.6735) (-8.0875, -10.964) (-7.4965, -11.2156) (-6.9894, -11.3405) (-6.5947, -11.3892) (-6.3253, -11.4) (-6.189, -11.4) knots 0 0 0 0 0 0 0.2 0.4 0.6 0.8 1 1 1 1 1 1
  line L68 (9.2055, -9.7365) -> (8.8184, -10.3617)
  line L69 (6.5567, -11.4) -> (5.8214, -11.4)
  line L70 (-9.2055, -9.7365) -> (-8.8184, -10.3617)
  line L71 (-6.5567, -11.4) -> (-5.8214, -11.4)
  line L72 (-5.45, -16.7) -> (5.45, -16.7)
  line L73 (5.45, -16.7) -> (5.45, -52.5)
  line L74 (5.45, -52.5) -> (-5.45, -52.5)
  line L75 (-5.45, -52.5) -> (-5.45, -16.7)
  line L76 (-5.45, -16.7) -> (5.45, -52.5) construction
  line L77 (5.45, -16.7) -> (-5.45, -52.5) construction
  line L78 (-5.45, -23.1541) -> (-4.312, -16.7)
  line L79 (-5.45, -23.1541) -> (0.7741, -23.1541) construction
  line L80 (-5.45, -46.0459) -> (-4.312, -52.5)
  line L81 (-5.45, -46.0459) -> (1.3736, -46.0459) construction
  line L82 (-4.312, -16.7) -> (-4.312, -52.5) construction
  line L83 (5.45, -46.0459) -> (4.312, -52.5)
  line L84 (5.45, -23.1541) -> (4.312, -16.7)
  line L85 (-20.2, -84.2434) -> (-20.2, -102.0248)
  line L86 (0, 18) -> (5, 18)
  line L87 (21.55, 15.05) -> (9.313, 15.05)
  arc A89 (5, 18) -> (9.313, 15.05) centre (9.313, 19.6778) ccw
  arc A90 (-9.313, 15.05) -> (-5, 18) centre (-9.313, 19.6778) ccw
  line L88 (-21.55, 15.05) -> (-9.313, 15.05)
  line L89 (0, 18) -> (-5, 18)
  line L90 (-15, -73.65) -> (-15, -103.65) construction
  circle A91 centre (-15, -103.65) radius 1.5
  circle A92 centre (-11.5, -118.65) radius 1.5
  circle A93 centre (-11.5, -118.65) radius 4.5
  line L91 (-15.7286, -120.1891) -> (-19.5733, -109.626)
  line L92 (-15.7286, -120.1891) -> (-5.1118, -120.1891) construction
  line L93 (-19.5733, -109.626) -> (-20.2, -102.0248)
  line L94 (0, -116) -> (-7.863, -116)
  line L95 (20.2, -84.2434) -> (20.2, -102.0248)
  circle A94 centre (15, -103.65) radius 1.5
  circle A95 centre (11.5, -118.65) radius 1.5
  line L96 (19.5733, -109.626) -> (20.2, -102.0248)
  line L97 (15.7286, -120.1891) -> (5.1118, -120.1891) construction
  line L98 (15.7286, -120.1891) -> (19.5733, -109.626)
  line L99 (0, -116) -> (7.863, -116)
  circle A96 centre (11.5, -118.65) radius 4.5
  line L100 (0, 44.45) -> (0, -156.9165) construction
  line L101 (27.3521, -87.3046) -> (20.2, -84.2434)
  point P0 (0, 44.45)
  point P1 (0, -34.6)
  point P2 (0, -34.6)
  point P3 (6.4, -82.51)
  point P4 (15, -103.65)
  dimension "d1" = 6.75
  dimension "d2" = 3
  dimension "d3" = 20
  dimension "d4" = 20
  dimension "d5" = 3
  dimension "d6" = 1.3
  dimension "d7" = 10.9
  dimension "d8" = 35.8
  dimension "d9" = 80
  dimension "d10" = 80
  dimension "d12" = 20.2
  dimension "d13" = 5
  dimension "d14" = 18
  dimension "d15" = 30
  dimension "d16" = 15
  dimension "d17" = 11.5
  dimension "d18" = 9
  dimension "d19" = 110
  dimension "d20" = 55
  constraint midpoint L55 origin
  constraint concentric A11 A75
  constraint concentric A23 A76
  constraint concentric A16 A77
  constraint concentric A7 A78
  constraint equal A77 A78
  constraint equal A76 A77
  constraint equal A75 A76
  constraint concentric A1 A79
  constraint concentric A0 A80
  constraint concentric A8 A81
  constraint concentric A17 A82
  constraint equal A81 A82
  constraint equal A80 A81
  constraint equal A79 A80
  constraint coincident A1.centre A79.centre
  constraint coincident A8.centre A81.centre
  constraint horizontal L59
  constraint perpendicular L59 L60
  constraint parallel L59 L61
  constraint parallel L60 L62
  constraint coincident L63 P2
  constraint coincident L64 P2
  constraint midpoint L58 P2
  constraint coincident L59.start L62.end
  constraint coincident L59.end L60.start
  constraint coincident L60.end L61.start
  constraint coincident L61.end L62.start
  constraint equal A85 A86
  constraint equal A84 A85
  constraint equal A83 A84
  constraint concentric A20 A87
  constraint concentric A4 A88
  constraint equal A87 A88
  constraint equal A81 A87
  constraint coincident P0 L66.start
  constraint perpendicular L59 L66
  constraint midpoint L57.end L68
  constraint midpoint L65.start L69
  constraint symmetric A14.start L66 A24.end
  constraint symmetric L57.end L66 L67.end
  constraint symmetric L65.start L66 L65.end
  constraint symmetric L66 L68.start L70.start
  constraint symmetric L66 L68.end L70.end
  constraint symmetric L66 L69.start L71.start
  constraint symmetric L66 L69.end L71.end
  constraint horizontal L72
  constraint perpendicular L72 L73
  constraint parallel L72 L74
  constraint parallel L73 L75
  constraint coincident L76 P2
  constraint coincident L77 P2
  constraint coincident P2 P1
  constraint horizontal L79
  constraint coincident L75 L78.start
  constraint horizontal L81
  constraint coincident L75 L80.start
  constraint coincident L74 L80.end
  constraint vertical L82
  constraint coincident L72 L78.end
  constraint symmetric L66 L78.start L84.start
  constraint symmetric L66 L78.end L84.end
  constraint symmetric L66 L80.start L83.start
  constraint symmetric L66 L80.end L83.end
  constraint parallel L66 L85
  constraint coincident L85 L7.end
  constraint coincident L66 L86.start
  constraint perpendicular L66 L86
  constraint tangent A21 L87
  constraint perpendicular L21 L87
  constraint horizontal L87
  constraint tangent L87 A89
  constraint symmetric L5.end L66 A63.start
  constraint symmetric L66 L86.start L89.start
  constraint symmetric L66 L86.end A90.end
  constraint symmetric L66 L87.end A90.start
  constraint symmetric L66 A89 A90
  constraint coincident A20.centre A87.centre
  constraint vertical L90
  constraint coincident L90.end A91.centre
  constraint equal A87 A91
  constraint equal A91 A92
  constraint concentric A92 A93
  constraint horizontal L92
  constraint coincident A93 L91.start
  constraint tangent A93 L91
  constraint coincident L66 L94.start
  constraint perpendicular L66 L94
  constraint coincident A93 L94.end
  constraint symmetric A70.centre L66 P3
  constraint symmetric P0 L66 L100.start
  constraint symmetric L100.end L66 L66.end
  constraint symmetric L66 L85.end L95.end
  constraint symmetric L66 L7.end L95.start
  constraint symmetric L66 L90.end P4
  constraint symmetric L66 A91 A94
  constraint symmetric L66 A92 A95
  constraint symmetric L66 A93 A96
  constraint symmetric L66 L91.start L97.start
  constraint symmetric L66 L91.end L96.start
  constraint symmetric L66 L92.end L97.end
  constraint symmetric L66 L94.start L99.start
  constraint symmetric L66 L94.end L99.end
  constraint symmetric L7.start L66 A9.start
  measures "d1" diameter of A75
  measures "d2" diameter of A79
  measures "d3" distance of L60.end L61.end
  measures "d4" distance of L59.end L60.end
  measures "d5" diameter of A83
  measures "d7" distance of L73.end L74.end
  measures "d8" distance of L72.end L73.end
  measures "d9" angle of L78 L79
  measures "d10" angle of L80 L81
  measures "d12" distance of L66 L85
  measures "d13" distance of L86.start L86.end
  measures "d14" distance of L55 L86
  measures "d15" distance of A20.centre L90.end
  measures "d16" vertical distance of L90.end A92.centre
  measures "d17" distance of L66 A92.centre
  measures "d18" diameter of A93
  measures "d19" angle of L91 L92
  measures "d20" distance of L47 L94
extrude "Extrude1" add sketch "Sketch1" along normal blind 2 contours L0 L1 L2 L3 A3 L5 A9 A11 L7 A13 L10 A16 L12 A23 L48 L50 A65 A67 A68 A69 A71 A72 L56 L85 L86 L87 A89 A90 L88 L89 A93 L91 L93 L94 L95 L96 L98 L99 A96 L101 | A96 | A93 | L72 L75 L78 | L72 L73 L84 | L74 L75 L80 | L73 L74 L83
fillet "Fillet1" radius 2 2 edges at (-20.2, -84.2434, 1) (20.2, -84.2434, 1)
fillet "Fillet2" radius 4 2 edges at (7.863, -116, 1) (-7.863, -116, 1)
fillet "Fillet3" radius 10 4 edges at (-19.5733, -109.626, 1) (-20.2, -102.0248, 1) (19.5733, -109.626, 1) (20.2, -102.0248, 1)
fillet "Fillet4" radius 1 4 edges at (-4.312, -16.7, 1) (4.312, -16.7, 1) (4.312, -52.5, 1) (-4.312, -52.5, 1)
fillet "Fillet5" radius 10 4 edges at (-5.45, -23.1541, 1) (5.45, -23.1541, 1) (5.45, -46.0459, 1) (-5.45, -46.0459, 1)